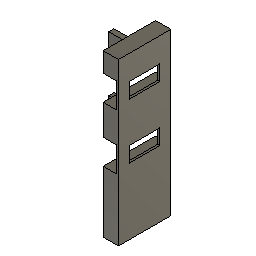
pegboard_mount_bracket (Autodesk Fusion 360 design; units mm, degrees)
part number: 2026-09-04-11-03-25-391
Autodesk Fusion 360 part; units mm, degrees
sketch "Plate" plane through (0, 0, 0) normal (0, 1, 0) x (1, 0, 0)
  line L0 (0, 0) -> (7, 0)
  line L1 (7, 0) -> (7, -74)
  line L2 (7, -74) -> (0, -74)
  line L3 (0, -74) -> (0, 0)
extrude "Plate (1)" add sketch "Plate" along normal mid plane 24
sketch "Hook profile" plane through (0, 0, 0) normal (0, 1, 0) x (1, 0, 0)
  line L0 (0, -72) -> (-8.3, -72)
  line L1 (-8.3, -72) -> (-8.3, -55)
  line L2 (-8.3, -55) -> (-5.3, -55)
  line L3 (-5.3, -55) -> (-3.8, -56.5)
  line L4 (-3.8, -56.5) -> (-3.8, -67)
  line L5 (-3.8, -67) -> (0, -67)
  line L6 (0, -67) -> (0, -72)
  dimension "d20" = 72
  dimension "d21" = 8.3
  dimension "d22" = 3.8
  dimension "d23" = 5
  dimension "d24" = 10.5
  dimension "d25" = 1.5
  dimension "d26" = 1.5
  constraint horizontal L0
  constraint horizontal L2
  constraint horizontal L5
  constraint vertical L1
  constraint vertical L4
  constraint vertical L6
  constraint coincident origin L6
  measures "d20" vertical distance of origin L0.start
  measures "d21" horizontal distance of L0.start L0.end
  measures "d22" horizontal distance of L4.end L5.end
  measures "d23" vertical distance of L0.start L5.end
  measures "d24" vertical distance of L3.end L4.end
  measures "d25" horizontal distance of L2.end L3.end
  measures "d26" vertical distance of L2.end L3.end
extrude "Hook profile (1)" add sketch "Hook profile" along normal mid plane 2.4
pattern_linear "Hook rows" count 2 spacing 25.4 along (0, 0, -1) count 3 spacing 0 along (0, 0, 1) of "Hook profile (1)"
sketch "Nut tracks" plane through (0, 0, 0) normal (0, 1, 0) x (1, 0, 0)
  line L0 (0, -53.545) -> (6, -53.545)
  line L1 (6, -53.545) -> (6, -65.055)
  line L2 (6, -65.055) -> (0, -65.055)
  line L3 (0, -65.055) -> (0, -53.545)
  line L4 (0, -28.145) -> (6, -28.145)
  line L5 (6, -28.145) -> (6, -39.655)
  line L6 (6, -39.655) -> (0, -39.655)
  line L7 (0, -39.655) -> (0, -28.145)
extrude "Nut tracks (1)" cut sketch "Nut tracks" along normal mid plane 34
sketch "Bolt slots" plane through (0, 0, 0) normal (0, 1, 0) x (1, 0, 0)
  line L0 (-1, -55.8) -> (8, -55.8)
  line L1 (8, -55.8) -> (8, -62.8)
  line L2 (8, -62.8) -> (-1, -62.8)
  line L3 (-1, -62.8) -> (-1, -55.8)
  line L4 (-1, -30.4) -> (8, -30.4)
  line L5 (8, -30.4) -> (8, -37.4)
  line L6 (8, -37.4) -> (-1, -37.4)
  line L7 (-1, -37.4) -> (-1, -30.4)
extrude "Bolt slots (1)" cut sketch "Bolt slots" along normal mid plane 14
equation "bracketWidth = 24.0 mm" comment "drives the model; safe to edit live in Fusion"
equation "hookTabWidth = 2.4 mm" comment "drives the model; safe to edit live in Fusion"
equation "slotPitchVertical = 25.4 mm" comment "drives the model; safe to edit live in Fusion"
equation "faceMetalThickness = 2.0 mm" comment "drives the model; safe to edit live in Fusion"
equation "hookThroat = faceMetalThickness + 1.8 mm" comment "drives the model; safe to edit live in Fusion"
equation "hookNeckHeight = 5.0 mm" comment "drives the model; safe to edit live in Fusion"
equation "hookLipThickness = 4.5 mm" comment "drives the model; safe to edit live in Fusion"
equation "hookLipDrop = 12.0 mm" comment "drives the model; safe to edit live in Fusion"
equation "hookLipChamfer = 1.5 mm" comment "drives the model; safe to edit live in Fusion"
equation "topHookNeckTop = 72.0 mm" comment "drives the model; safe to edit live in Fusion"
equation "hookRows = 2" comment "drives the model; safe to edit live in Fusion"
equation "plateThickness = 7.0 mm" comment "reference only â edit scripts/build_pegboard_bracket.py and rebuild"
equation "plateHeight = 74.0 mm" comment "reference only â edit scripts/build_pegboard_bracket.py and rebuild"
equation "boltSlotHeight = 7.0 mm" comment "reference only â edit scripts/build_pegboard_bracket.py and rebuild"
equation "boltSlotLength = 14.0 mm" comment "reference only â edit scripts/build_pegboard_bracket.py and rebuild"
equation "nutTrackHeight = 11.51 mm" comment "reference only â edit scripts/build_pegboard_bracket.py and rebuild"
equation "nutTrackDepth = 6.0 mm" comment "reference only â edit scripts/build_pegboard_bracket.py and rebuild"
equation "d18 = bracketWidth"
equation "d20 = topHookNeckTop"
equation "d21 = hookThroat + hookLipThickness"
equation "d22 = hookThroat"
equation "d23 = hookNeckHeight"
equation "d24 = hookLipDrop - hookLipChamfer"
equation "d25 = hookLipChamfer"
equation "d26 = hookLipChamfer"
equation "d27 = hookTabWidth"
equation "d29 = hookRows"
equation "d31 = -slotPitchVertical"
equation "d33 = bracketWidth + 10 mm"
named bodies: "pegboard_mount_bracket"
